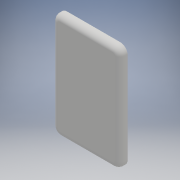
# Autodesk Inventor part: Test
Saved by Autodesk Inventor 2017 (Build 210142000, 142)
## iProperties
Created: 2018-08-10
Part Number: Test
Material: Generic
Document SubType Name: Modeling
Designer: intelsath
Density: 1 g/cm^3
Appearance: Default
Author: intelsath
Autodesk Inventor part; units mm, degrees
ref_plane "YZ Plane" through (0, 0, 0) normal (1, 0, 0) x (0, 1, 0)
ref_plane "XZ Plane" through (0, 0, 0) normal (0, 1, 0) x (-1, 0, 0)
ref_plane "XY Plane" through (0, 0, 0) normal (0, 0, 1) x (1, 0, 0)
sketch "Sketch1" plane through (0, 0, 0) normal (0, 1, 0) x (-1, 0, 0)
  line L0 (0, 0) -> (-9, 0)
  line L1 (-9, 0) -> (-9, -14)
  line L2 (-9, -14) -> (0, -14)
  line L3 (0, -14) -> (0, 0)
  dimension "d0" = 9
  dimension "d1" = 14
  constraints: 8 end point, 2 parallel, 1 horizontal, 1 perpendicular
  measures "d0" distance of L2.end L1.end
  measures "d1" distance of L1.end L0.end
extrude "Extrusion1" add sketch "Sketch1" along normal blind 1
fillet "Fillet1" radius 0.7 4 edges at (0, 0, -7) (4.5, 0, -14) (9, 0, -7) (4.5, 0, 0)
fillet "Fillet2" radius 1 8 edges at (0, 0.85, -14) (0.205, 0.205, -13.795) (8.795, 0.205, -13.795) (9, 0.85, -14) (8.795, 0.205, -0.205) (9, 0.85, 0) (0, 0.85, 0) (0.205, 0.205, -0.205)
body "Solid1"
